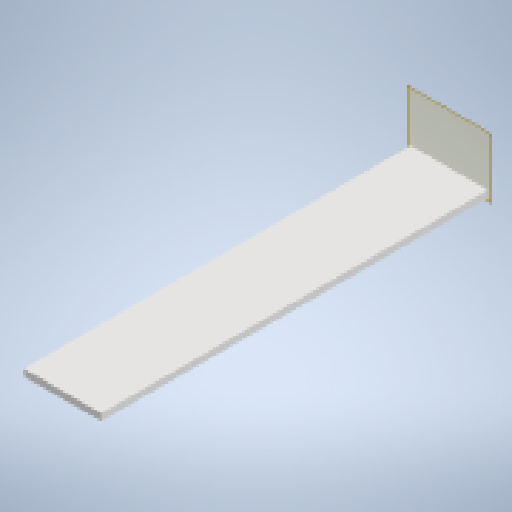
# Autodesk Inventor part: base-back
Saved by Autodesk Inventor 2023 (Build 270158030, 158C)
## iProperties
Created: 2024-09-10
Part Number: base-back
Material: Generic
Document SubType Name: Modeling
Designer: Imogen Heard
Density: 1 g/cm^3
Appearance: Default
Author: Imogen Heard
Autodesk Inventor part; units mm, degrees
ref_plane "YZ Plane" through (0, 0, 0) normal (1, 0, 0) x (0, 1, 0)
ref_plane "XZ Plane" through (0, 0, 0) normal (0, 1, 0) x (-1, 0, 0)
ref_plane "XY Plane" through (0, 0, 0) normal (0, 0, 1) x (1, 0, 0)
ref_plane "Work Plane1" through (0, 0, 0) normal (0, 0, 1) x (1, 0, 0)
sketch "Sketch1" plane through (0, 0, 0) normal (0, 0, 1) x (1, 0, 0)
  line L0 (-270, -89.7729) -> (-720, -193.6636) projected
  line L1 (-720, -193.6636) -> (-708.7524, -242.3821) projected
  line L2 (-708.7524, -242.3821) -> (-264.3032, -139.7729) projected
  line L3 (-200, -139.7729) -> (-264.3032, -139.7729) projected
  line L4 (-200, -91.2956) -> (-200, -139.7729) projected
  line L5 (130, 139.7729) -> (-200, -91.2956) projected
  line L6 (130, -104.7729) -> (130, 139.7729) projected
  line L7 (200, -104.7729) -> (130, -104.7729) projected
  line L8 (200, 275.2271) -> (200, -104.7729) projected
  line L9 (130, 275.2271) -> (200, 275.2271) projected
  line L10 (130, 225.2271) -> (130, 275.2271) projected
  line L11 (-200, -5.8414) -> (130, 225.2271) projected
  line L12 (-200, 310.2271) -> (-200, -5.8414) projected
  line L13 (-270, 310.2271) -> (-200, 310.2271) projected
  line L14 (-270, -89.7729) -> (-270, 310.2271) projected
  arc A0 (-230, -34.7729) -> (-240, -24.7729) centre (-240, -34.7729) ccw projected
  line L15 (-230, -34.7729) -> (-230, -74.7729) projected
  arc A1 (-240, -84.7729) -> (-230, -74.7729) centre (-240, -74.7729) ccw projected
  line L16 (-240, -84.7729) -> (-250, -84.7729) projected
  arc A2 (-260, -74.7729) -> (-250, -84.7729) centre (-250, -74.7729) ccw projected
  line L17 (-260, -74.7729) -> (-260, -34.7729) projected
  arc A3 (-250, -24.7729) -> (-260, -34.7729) centre (-250, -34.7729) ccw projected
  line L18 (-250, -24.7729) -> (-240, -24.7729) projected
  arc A4 (-230, 225.2271) -> (-240, 235.2271) centre (-240, 225.2271) ccw projected
  line L19 (-230, 225.2271) -> (-230, 185.2271) projected
  arc A5 (-240, 175.2271) -> (-230, 185.2271) centre (-240, 185.2271) ccw projected
  line L20 (-240, 175.2271) -> (-250, 175.2271) projected
  arc A6 (-260, 185.2271) -> (-250, 175.2271) centre (-250, 185.2271) ccw projected
  line L21 (-260, 185.2271) -> (-260, 225.2271) projected
  arc A7 (-250, 235.2271) -> (-260, 225.2271) centre (-250, 225.2271) ccw projected
  line L22 (-250, 235.2271) -> (-240, 235.2271) projected
  arc A8 (-230, 160.2271) -> (-240, 170.2271) centre (-240, 160.2271) ccw projected
  line L23 (-230, 160.2271) -> (-230, 120.2271) projected
  arc A9 (-240, 110.2271) -> (-230, 120.2271) centre (-240, 120.2271) ccw projected
  line L24 (-240, 110.2271) -> (-250, 110.2271) projected
  arc A10 (-260, 120.2271) -> (-250, 110.2271) centre (-250, 120.2271) ccw projected
  line L25 (-260, 120.2271) -> (-260, 160.2271) projected
  arc A11 (-250, 170.2271) -> (-260, 160.2271) centre (-250, 160.2271) ccw projected
  line L26 (-250, 170.2271) -> (-240, 170.2271) projected
  arc A12 (-230, 30.2271) -> (-240, 40.2271) centre (-240, 30.2271) ccw projected
  line L27 (-230, 30.2271) -> (-230, -9.7729) projected
  arc A13 (-240, -19.7729) -> (-230, -9.7729) centre (-240, -9.7729) ccw projected
  line L28 (-240, -19.7729) -> (-250, -19.7729) projected
  arc A14 (-260, -9.7729) -> (-250, -19.7729) centre (-250, -9.7729) ccw projected
  line L29 (-260, -9.7729) -> (-260, 30.2271) projected
  arc A15 (-250, 40.2271) -> (-260, 30.2271) centre (-250, 30.2271) ccw projected
  line L30 (-250, 40.2271) -> (-240, 40.2271) projected
  arc A16 (-230, 290.2271) -> (-240, 300.2271) centre (-240, 290.2271) ccw projected
  line L31 (-230, 290.2271) -> (-230, 250.2271) projected
  arc A17 (-240, 240.2271) -> (-230, 250.2271) centre (-240, 250.2271) ccw projected
  line L32 (-240, 240.2271) -> (-250, 240.2271) projected
  arc A18 (-260, 250.2271) -> (-250, 240.2271) centre (-250, 250.2271) ccw projected
  line L33 (-260, 250.2271) -> (-260, 290.2271) projected
  arc A19 (-250, 300.2271) -> (-260, 290.2271) centre (-250, 290.2271) ccw projected
  line L34 (-250, 300.2271) -> (-240, 300.2271) projected
  arc A20 (-230, 95.2271) -> (-240, 105.2271) centre (-240, 95.2271) ccw projected
  line L35 (-230, 95.2271) -> (-230, 55.2271) projected
  arc A21 (-240, 45.2271) -> (-230, 55.2271) centre (-240, 55.2271) ccw projected
  line L36 (-240, 45.2271) -> (-250, 45.2271) projected
  arc A22 (-260, 55.2271) -> (-250, 45.2271) centre (-250, 55.2271) ccw projected
  line L37 (-260, 55.2271) -> (-260, 95.2271) projected
  arc A23 (-250, 105.2271) -> (-260, 95.2271) centre (-250, 95.2271) ccw projected
  line L38 (-250, 105.2271) -> (-240, 105.2271) projected
  line L39 (-200, -139.7729) -> (-200, -91.2956) projected
  line L40 (-200, -139.7729) -> (200, -139.7729) projected
  line L41 (200, -139.7729) -> (200, -104.7729) projected
  line L42 (130, -104.7729) -> (200, -104.7729) projected
  line L43 (130, 139.7729) -> (130, -104.7729) projected
  line L44 (-200, -91.2956) -> (130, 139.7729) projected
  line L45 (200, 275.2271) -> (200, 310.2271) projected
  line L46 (200, 310.2271) -> (-200, 310.2271) projected
  line L47 (-200, -5.8414) -> (-200, 310.2271) projected
  line L48 (130, 225.2271) -> (-200, -5.8414) projected
  line L49 (130, 275.2271) -> (130, 225.2271) projected
  line L50 (200, 275.2271) -> (130, 275.2271) projected
  line L51 (200, -104.7729) -> (-200, -104.7729)
  line L52 (-200, -104.7729) -> (-200, -139.7729)
  line L53 (-200, -139.7729) -> (200, -139.7729)
  line L54 (200, -139.7729) -> (200, -104.7729)
  point P0 (0, 0)
  point P1 (-200, -104.7729)
  constraints: 8 end point, 2 parallel, 1 horizontal, 1 perpendicular
extrude "Extrusion1" add sketch "Sketch1" along normal blind 2030 contours L4 L51 L7 L41 L40
